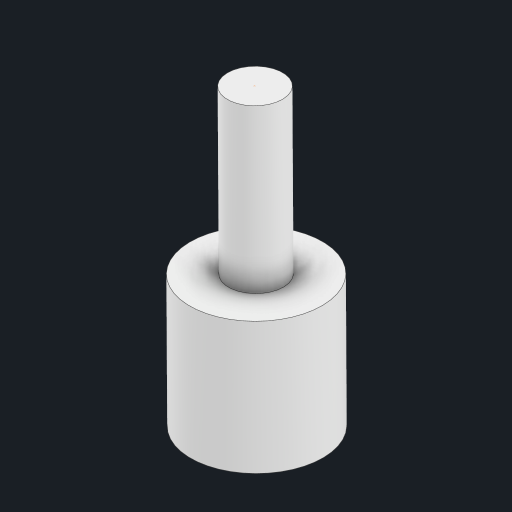
# Autodesk Inventor part: base
Saved by Autodesk Inventor 2023 (Build 270158000, 158)
## iProperties
Created: 2024-02-21
Part Number: base
Material: ABS Plastic
Document SubType Name: Modeling
Designer: valer
Density: 1.06 g/cm^3
Appearance: Smooth - White
Mass: 27291.1 g
Surface Area: 5694.14 cm^2
Volume: 25746.3 cm^3
Author: valer
Autodesk Inventor part; units mm, degrees
ref_plane "YZ Plane" through (0, 0, 0) normal (1, 0, 0) x (0, 1, 0)
ref_plane "XZ Plane" through (0, 0, 0) normal (0, 1, 0) x (-1, 0, 0)
ref_plane "XY Plane" through (0, 0, 0) normal (0, 0, 1) x (1, 0, 0)
sketch "BaseProfile" plane through (0, 0, 0) normal (0, 0, 1) x (1, 0, 0)
  circle A0 centre (0, 0) radius 150
  dimension "d0" = 300
  constraints: 1 centre point, 1 coincident
  measures "d0" diameter of A0
extrude "Base" add sketch "BaseProfile" along normal blind 300
sketch "Joint" plane through (0, 0, 300) normal (0, 0, 1) x (1, 0, 0)
  circle A0 centre (0, 0) radius 150 projected
  circle A1 centre (0, 0) radius 150 projected
  circle A2 centre (0, 0) radius 62.5
  dimension "d3" = 125
  constraints: 1 centre point, 1 coincident
  measures "d3" diameter of A2
extrude "JointAxis" add sketch "Joint" along normal blind 370 contours A2
sketch "Connector" plane through (0, 0, 670) normal (0, 0, 1) x (1, 0, 0)
  point P0 (0, 0)
body "Solid1"
